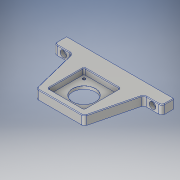
# Autodesk Inventor part: Y-Motorhalter
Saved by Autodesk Inventor 2019 (Build 230136000, 136)
## iProperties
Created: 2021-04-25
Part Number: Y-Motorhalter
Material: Aluminium 6061
Document SubType Name: Modeling
Designer: Michael Sumper
Density: 2.7 g/cm^3
Appearance: Aluminium - flach
Mass: 349.523 g
Surface Area: 322.582 cm^2
Volume: 129.453 cm^3
Stock Number: 0
Author: Michael Sumper
Autodesk Inventor part; units mm, degrees
ref_plane "YZ Plane" through (0, 0, 0) normal (1, 0, 0) x (0, 1, 0)
ref_plane "XZ Plane" through (0, 0, 0) normal (0, 1, 0) x (-1, 0, 0)
ref_plane "XY Plane" through (0, 0, 0) normal (0, 0, 1) x (1, 0, 0)
sketch "Skizze1" plane through (0, 0, 0) normal (0, 1, 0) x (-1, 0, 0)
  circle A0 centre (0, 0) radius 19.1
  line L0 (23.5, 23.5) -> (-23.5, 23.5) construction
  line L1 (-23.5, 23.5) -> (-23.5, -23.5) construction
  line L2 (-23.5, -23.5) -> (23.5, -23.5) construction
  line L3 (23.5, -23.5) -> (23.5, 23.5) construction
  line L4 (23.5, 23.5) -> (-23.5, -23.5) construction
  line L5 (-23.5, 23.5) -> (23.5, -23.5) construction
  circle A1 centre (23.5, 23.5) radius 2.2
  circle A2 centre (23.5, -23.5) radius 2.2
  circle A3 centre (-23.5, -23.5) radius 2.2
  circle A4 centre (-23.5, 23.5) radius 2.2
  line L6 (30, 30) -> (-30, 30)
  line L7 (-30, 30) -> (-30, -30)
  line L8 (-30, -30) -> (30, -30)
  line L9 (30, -30) -> (30, 30)
  line L10 (30, 30) -> (-30, -30) construction
  line L11 (-30, 30) -> (30, -30) construction
  line L12 (40, 40) -> (-40, 40)
  line L13 (-40, 40) -> (-40, -40) construction
  line L14 (-40, -40) -> (40, -40) construction
  line L15 (40, -40) -> (40, 40) construction
  line L16 (40, 40) -> (-40, -40) construction
  line L17 (-40, 40) -> (40, -40) construction
  line L18 (0, -40) -> (0, -60) construction
  line L19 (0, -40) -> (20, -40) construction
  line L20 (0, -60) -> (-90, -60)
  line L21 (-90, -60) -> (-90, -40)
  line L22 (-90, -40) -> (-60, -40)
  line L23 (-60, -40) -> (-40, 40)
  line L24 (0, -60) -> (90, -60)
  line L25 (0, -60) -> (90, -60) construction
  line L26 (90, -60) -> (90, -40)
  line L27 (90, -40) -> (60, -40)
  line L28 (60, -40) -> (40, 40)
  dimension "d0" = 38.2
  dimension "d1" = 47
  dimension "d2" = 47
  dimension "d3" = 4.4
  dimension "d4" = 4.4
  dimension "d5" = 4.4
  dimension "d6" = 4.4
  dimension "d7" = 60
  dimension "d8" = 60
  dimension "d9" = 80
  dimension "d10" = 80
  dimension "d11" = 20
  dimension "d12" = 90
  dimension "d13" = 90
  dimension "d14" = 20
  dimension "d15" = 30
  dimension "d16" = 90
  dimension "d17" = 0
  dimension "d18" = 20
  dimension "d19" = 30
  constraints: 58 end point, 7 midpoint, 7 parallel, 6 horizontal, 5 centre point, 5 coincident, 5 perpendicular, 2 equal length, 2 point on line, 1 vertical
  measures "d0" diameter of A0
  measures "d1" distance of L2.end L1.end
  measures "d2" distance of L1.end L0.end
  measures "d3" diameter of A1
  measures "d4" diameter of A2
  measures "d5" diameter of A3
  measures "d6" diameter of A4
  measures "d7" distance of L8.end L7.end
  measures "d8" distance of L7.end L6.end
  measures "d9" distance of L14.end L13.end
  measures "d10" distance of L13.end L12.end
  measures "d11" distance of L18.start L18.end
  measures "d12" angle of L18 L19
  measures "d13" distance of L18.end L20.end
  measures "d14" distance of L20.end L21.end
  measures "d15" distance of L21.end L22.end
  measures "d16" distance of L18.end L24.end
  measures "d17" distance between parallel lines of L24 L25
  measures "d18" distance of L24.end L26.end
  measures "d19" distance of L26.end L27.end
extrude "Extrusion1" add sketch "Skizze1" along normal blind 5 contours L9 L8 L7 L6
extrude "Extrusion2" add sketch "Skizze1" along normal blind 15 contours L28 L27 L26 L24 L20 L21 L22 L23 L12
fillet "Rundung1" radius 5 6 edges at (-90, 7.5, -40) (-60, 7.5, -40) (60, 7.5, -40) (90, 7.5, -40) (40, 7.5, 40) (-40, 7.5, 40)
fillet "Rundung2" radius 2 4 edges at (-30, 10, -30) (30, 10, -30) (30, 10, 30) (-30, 10, 30)
chamfer "Fase1" distance 1 angle 45 21 edges at (-74.4519, 15, -40) (-60.8268, 15, -38.941) (-50, 15, 0) (-39.1732, 15, 38.941) (0, 15, 40) (39.1732, 15, 38.941) (50, 15, 0) (60.8268, 15, -38.941) (74.4519, 15, -40) (88.5355, 15, -41.4645) (90, 15, -52.5) (-88.5355, 15, -41.4645) (-90, 15, -52.5) (-30, 15, 0) (-29.4142, 15, -29.4142) (0, 15, -30) (29.4142, 15, -29.4142) (30, 15, 0) (29.4142, 15, 29.4142) (0, 15, 30) (-29.4142, 15, 29.4142)
chamfer "Fase2" distance 0.1 angle 45 5 edges at (-21.3, 5, -23.5) (25.7, 5, -23.5) (19.1, 5, 0) (25.7, 5, 23.5) (-21.3, 5, 23.5)
thread "Gewinde1" size "M5x0.8" class "6H" standard "ISO Metric profile" full length
thread "Gewinde2" size "M5x0.8" class "6H" standard "ISO Metric profile" full length
sketch "Skizze2" plane through (-85, 0, -40) normal (0, 0, 1) x (1, 0, 0)
  line L0 (0, 0) -> (0, 14) construction
  line L1 (0, 14) -> (0, 15) construction
  line L2 (21.0961, 15) -> (0, 15) construction
  line L3 (21.0961, 14) -> (21.0961, 15) construction
  line L4 (21.0961, 14) -> (21.0961, 0) construction
  line L5 (0, 0) -> (21.0961, 0) construction
  line L6 (148.9039, 0) -> (148.9039, 14) construction
  line L7 (148.9039, 14) -> (148.9039, 15) construction
  line L8 (170, 15) -> (148.9039, 15) construction
  line L9 (170, 14) -> (170, 15) construction
  line L10 (170, 14) -> (170, 0) construction
  line L11 (148.9039, 0) -> (170, 0) construction
  line L12 (0, 15) -> (21.0961, 0)
  line L13 (21.0961, 15) -> (0, 0)
  line L14 (175, 0) -> (170, 0) construction
  line L15 (148.9039, 15) -> (170, 0)
  line L16 (170, 15) -> (148.9039, 0)
  point P0 (85, 0)
  constraints: 8 end point, 1 parallel
sketch "Skizze3" plane through (-85, 0, -40) normal (0, 0, 1) x (1, 0, 0)
  point P0 (85, 0)
  point P1 (10.548, 7.4957)
  point P2 (159.4529, 7.4965)
hole "Bohrung1" at (-74.452, 7.4957, -40) at (74.4529, 7.4965, -40) direction (0, 0, -1) diameter 6.6 end through all counterbore diameter 11 counterbore depth 6 clearance for "Innensechskantkopfschraube" size "M6" standard "ANSI Metrisches M Profil"
thread "Gewinde3" size "M5x0.8" class "6H" standard "ISO Metric profile" full length
thread "Gewinde4" size "M5x0.8" class "6H" standard "ISO Metric profile" full length
